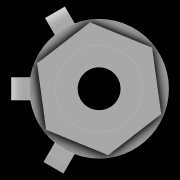
# Autodesk Inventor part: fishman-jack
Saved by Autodesk Inventor 2020 (Build 240168000, 168)
## iProperties
Created: 2020-01-01
Part Number: fishman-jack
Material: Generic
Document SubType Name: Modeling
Designer: valer
Density: 1 g/cm^3
Appearance: Default
Author: valer
Autodesk Inventor part; units mm, degrees
note: some values were not read from the file. Chosen so that the rebuilt part matches the saved one: bend side of "Bend Part2"; bend side of "Bend Part3".
ref_plane "YZ Plane" through (0, 0, 0) normal (1, 0, 0) x (0, 1, 0)
ref_plane "XZ Plane" through (0, 0, 0) normal (0, 1, 0) x (-1, 0, 0)
ref_plane "XY Plane" through (0, 0, 0) normal (0, 0, 1) x (1, 0, 0)
sketch "Fishman1/4Jack" plane through (0, 0, 0) normal (0, 0, 1) x (1, 0, 0)
  circle A0 centre (0, 0) radius 10.16
  line L0 (-10.3198, 14.5724) -> (-7.4602, 16.2234)
  line L1 (-7.4602, 16.2234) -> (-2.3802, 7.4246)
  line L2 (-2.3802, 7.4246) -> (-5.2398, 5.7736)
  line L3 (-5.2398, 5.7736) -> (-10.3198, 14.5724)
  line L4 (-17.78, 1.651) -> (-7.62, 1.651)
  line L5 (-7.62, 1.651) -> (-7.62, -1.651)
  line L6 (-7.62, -1.651) -> (-17.78, -1.651)
  line L7 (-17.78, -1.651) -> (-17.78, 1.651)
  line L8 (-10.3198, -14.5724) -> (-7.4602, -16.2234)
  line L9 (-7.4602, -16.2234) -> (-2.3802, -7.4246)
  line L10 (-2.3802, -7.4246) -> (-5.2398, -5.7736)
  line L11 (-5.2398, -5.7736) -> (-10.3198, -14.5724)
  circle A1 centre (0, 0) radius 3.175
  line L12 (-8.89, 15.3979) -> (0, 0) construction
  line L13 (-17.78, 0) -> (0, 0) construction
  line L14 (0, 0) -> (-8.89, -15.3979) construction
  circle A2 centre (-8.255, 14.2981) radius 0.635
  circle A3 centre (-16.51, 0) radius 0.635
  circle A4 centre (-8.255, -14.2981) radius 0.635
  point P0 (-3.81, 6.5991)
  point P1 (-3.81, -6.5991)
  point P2 (-3.5827, -9.5074)
  point P3 (-6.4423, -7.8564)
  point P4 (-10.025, -1.651)
  point P5 (-10.025, 1.651)
  point P6 (-6.4423, 7.8564)
  point P7 (-3.5827, 9.5074)
  dimension "d37" = 20.32
  dimension "d38" = 60
  dimension "d39" = 60
  dimension "d60" = 17.78
  dimension "d61" = 3.302
  dimension "d62" = 6.35
  dimension "d63" = 10.16
  dimension "d129" = 1.27
  dimension "d130" = 1.27
  dimension "d131" = 1.27
  dimension "d132" = 1.27
  constraints: 30 end point, 6 equal length, 6 parallel, 5 centre point, 5 midpoint, 5 point on line, 3 perpendicular, 2 coincident, 2 equal radius, 2 horizontal
  measures "d37" diameter of A0
  measures "d38" angle of L12 L13
  measures "d39" angle of L13 L14
  measures "d60" distance of L12.start L14.start
  measures "d61" distance of L3.end L1.start
  measures "d62" diameter of A1
  measures "d63" distance between parallel lines of L0 L2
  measures "d129" diameter of A2
  measures "d130" distance from line of L0 A2.centre
  measures "d131" distance from line of L7 A3.centre
  measures "d132" distance from line of L8 A4.centre
extrude "FishmanJackBodyFeature" add sketch "Fishman1/4Jack" along normal blind 1.27 contours A0 L9 L10 L11 L6 L5 L4 L3 L2 L1 | L1 L2 L3 A0 | A0 L11 L10 L9 | L4 L5 L6 A0 | A1
extrude "FishmanJackLegsFeature" add sketch "Fishman1/4Jack" along normal blind 1.27 contours A0 L3 L0 L1 | L9 L8 L11 A0 | A0 L6 L7 L4
fillet "FishmanJackLegFilletsFeature" radius 1.27 6 edges at (-10.3198, 14.5724, 0.635) (-7.4602, 16.2234, 0.635) (-17.78, 1.651, 0.635) (-17.78, -1.651, 0.635) (-7.4602, -16.2234, 0.635) (-10.3198, -14.5724, 0.635)
sketch "Sketch15" plane through (0, 0, 1.27) normal (0, 0, 1) x (1, 0, 0)
  circle A0 centre (0, 0) radius 6.35
  dimension "d134" = 12.7
  constraints: 1 centre point, 1 coincident
  measures "d134" diameter of A0
extrude "Extrusion10" add sketch "Sketch15" along normal blind 1.27
sketch "Sketch16" plane through (0, 0, 2.54) normal (0, 0, 1) x (1, 0, 0)
  circle A0 centre (0, 0) radius 10.16 projected
extrude "Extrusion11" add sketch "Sketch16" along normal blind 1.27
sketch "Sketch17" plane through (0, 0, 3.81) normal (0, 0, 1) x (1, 0, 0)
  circle A0 centre (0, 0) radius 6.35
  dimension "d139" = 12.7
  constraints: 1 centre point, 1 coincident
  measures "d139" diameter of A0
extrude "Extrusion12" add sketch "Sketch17" along normal blind 1.27
sketch "Sketch18" plane through (0, 0, 5.08) normal (0, 0, 1) x (1, 0, 0)
  circle A0 centre (0, 0) radius 10.16 projected
extrude "Extrusion13" add sketch "Sketch18" along normal blind 2.54
sketch "Sketch19" plane through (0, 0, 7.62) normal (0, 0, 1) x (1, 0, 0)
  circle A0 centre (0, 0) radius 3.175
  dimension "d144" = 6.35
  constraints: 1 centre point, 1 coincident
  measures "d144" diameter of A0
extrude "Extrusion14" cut sketch "Sketch19" against normal through all
sketch "Sketch20" plane through (0, 0, 7.62) normal (0, 0, 1) x (1, 0, 0)
  line L0 (7.7243, 5.9929) -> (9.0521, -3.693)
  line L1 (9.0521, -3.693) -> (1.3278, -9.6859)
  line L2 (1.3278, -9.6859) -> (-7.7243, -5.9929)
  line L3 (-7.7243, -5.9929) -> (-9.0521, 3.693)
  line L4 (-9.0521, 3.693) -> (-1.3278, 9.6859)
  line L5 (-1.3278, 9.6859) -> (7.7243, 5.9929)
  circle A0 centre (0, 0) radius 3.175 projected
  dimension "d147" = 8.4667
  constraints: 12 end point, 1 coincident, 13 other
  measures "d147" distance from line of L3 point (0, 0)
extrude "Extrusion15" add sketch "Sketch20" along normal blind 2.54
sketch "Sketch21" plane through (0, 0, 10.16) normal (0, 0, 1) x (1, 0, 0)
  circle A0 centre (0, 0) radius 3.175 projected
  circle A1 centre (0, 0) radius 6.35
  dimension "d150" = 12.7
  constraints: 1 centre point, 1 coincident
  measures "d150" diameter of A1
extrude "Extrusion16" add sketch "Sketch21" along normal blind 6.35
sketch "Sketch22" plane through (0, 0, 1.27) normal (0, 0, 1) x (1, 0, 0)
  line L0 (-9.6848, 13.4726) -> (-6.4423, 7.8564) projected
  line L1 (-7.101, 8.9973) -> (-4.2629, 10.6358)
  line L2 (-3.5827, 9.5074) -> (-6.8252, 15.1236) projected
  point P0 (0, 0)
  dimension "d153" = 1.3174
  constraints: 2 end point, 2 perpendicular, 1 point on line
  measures "d153" distance of L0.end L1.start
bend part "Bend Part1" radius 1.524 angle 90 line through (-7.101, 8.9973, 1.27) along (0.8660254, 0.5, 0) centre toward (0, 0, -1) moving side (-0.5, 0.8660254, 0) both sides no
sketch "Sketch23" plane through (0, 0, 1.27) normal (0, 0, 1) x (1, 0, 0)
  line L0 (-10.025, 1.651) -> (-16.51, 1.651) projected
  line L1 (-11.295, 1.651) -> (-11.295, -1.651)
  line L2 (-16.51, -1.651) -> (-10.025, -1.651) projected
  point P0 (0, 0)
  dimension "d156" = 1.27
  constraints: 2 end point, 2 point on line, 1 vertical
  measures "d156" distance from line of L1 L0.start
bend part "Bend Part2" radius 1.524 angle 90 line through (-11.295, 1.651, 1.27) along (0, -1, 0) centre toward (0, 0, -1) moving side (-1, 0, 0) both sides no
sketch "Sketch24" plane through (0, 0, 1.27) normal (0, 0, 1) x (1, 0, 0)
  line L0 (-6.4423, -7.8564) -> (-9.6848, -13.4726) projected
  line L1 (-7.3143, -9.3668) -> (-4.4547, -11.0178)
  line L2 (-6.8252, -15.1236) -> (-3.5827, -9.5074) projected
  point P0 (0, 0)
  dimension "d159" = 4.741
  constraints: 2 end point, 2 point on line, 1 perpendicular
  measures "d159" distance from line of L0.end L1
bend part "Bend Part3" radius 1.524 angle 90 line through (-7.3143, -9.3668, 1.27) along (0.8660254, -0.5, 0) centre toward (0, 0, -1) moving side (-0.5, -0.8660254, 0) both sides no
thread "Thread1" size "1/2-13 UNC" class "2A" standard "ANSI Unified Screw Threads" full length
body "Solid3"
